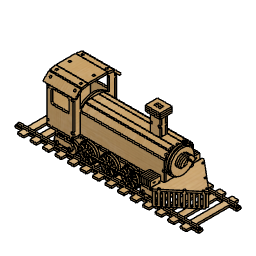
train-3D-model (Autodesk Fusion 360 design; units mm, degrees)
Autodesk Fusion 360 part; units mm, degrees
note: some values were not read from the file. Set by a fixed rule: which sketch regions a step uses.
(part 1 of 4)
sketch "Sketch1" plane through (0, 0, 0) normal (0, 1, 0) x (1, 0, 0)
  circle A0 centre (0, 0) radius 15
  line L0 (0, 0) -> (35, 0) construction
  circle A1 centre (35, 0) radius 15
  line L1 (0, 0) -> (-35, 0) construction
  circle A2 centre (-35, 0) radius 15
  line L2 (-33.5, -3) -> (-33.5, 3)
  line L3 (-33.5, 3) -> (-36.5, 3)
  line L4 (-36.5, 3) -> (-36.5, -3)
  line L5 (-36.5, -3) -> (-33.5, -3)
  line L6 (-1.5, -3) -> (-1.5, 3)
  line L7 (-1.5, 3) -> (1.5, 3)
  line L8 (1.5, 3) -> (1.5, -3)
  line L9 (1.5, -3) -> (-1.5, -3)
  line L10 (36.5, 3) -> (36.5, -3)
  line L11 (36.5, -3) -> (33.5, -3)
  line L12 (33.5, -3) -> (33.5, 3)
  line L13 (33.5, 3) -> (36.5, 3)
  circle A3 centre (81, 6) radius 9
  line L14 (35, 15) -> (81, 15) construction
  line L15 (35, 15) -> (61, 15) construction
  circle A4 centre (61, 6) radius 9
  line L16 (62.5, 3) -> (62.5, 9)
  line L17 (62.5, 9) -> (59.5, 9)
  line L18 (59.5, 9) -> (59.5, 3)
  line L19 (62.5, 3) -> (59.5, 3)
  line L20 (82.5, 3) -> (82.5, 9)
  line L21 (82.5, 9) -> (79.5, 9)
  line L22 (79.5, 9) -> (79.5, 3)
  line L23 (79.5, 3) -> (82.5, 3)
  circle A5 centre (-61, 6) radius 9
  circle A6 centre (-81, 6) radius 9
  line L24 (-62.5, 3) -> (-59.5, 3)
  line L25 (-59.5, 9) -> (-59.5, 3)
  line L26 (-62.5, 9) -> (-59.5, 9)
  line L27 (-62.5, 3) -> (-62.5, 9)
  line L28 (-79.5, 9) -> (-79.5, 3)
  line L29 (-79.5, 3) -> (-82.5, 3)
  line L30 (-82.5, 3) -> (-82.5, 9)
  line L31 (-82.5, 9) -> (-79.5, 9)
  dimension "d1" = 30
  dimension "d2" = 35
  dimension "d3" = 30
  dimension "d4" = 35
  dimension "d5" = 30
  dimension "d7" = 3
  dimension "d8" = 18
  dimension "d9" = 46
  dimension "d10" = 26
  dimension "d11" = 18
  dimension "d14" = 3
  dimension "d16" = 6
  dimension "d17" = 3
  constraint coincident A0.centre L0.start
  constraint horizontal L0
  constraint coincident L0.end A1.centre
  constraint parallel L0 L1
  constraint coincident L1.end A2.centre
  constraint perpendicular L1 L2
  constraint perpendicular L2 L3
  constraint perpendicular L3 L4
  constraint perpendicular L2 L5
  constraint coincident A1 L14.start
  constraint horizontal L14
  constraint tangent A1 L14
  constraint tangent A3 L14
  constraint coincident A3 L14.end
  constraint parallel L14 L15
  constraint tangent L15 A4
  constraint coincident L15.end A4
  constraint perpendicular L16 L17
  constraint perpendicular L17 L18
  constraint perpendicular L20 L21
  constraint perpendicular L21 L22
  constraint perpendicular L20 L23
  measures "d1" diameter of A0
  measures "d2" distance of A0.centre L0.end
  measures "d3" diameter of A1
  measures "d4" distance of A0.centre L1.end
  measures "d5" diameter of A2
  measures "d7" distance of L2.end L3.end
  measures "d8" diameter of A3
  measures "d9" distance of L14.start L14.end
  measures "d10" distance of L14.start L15.end
  measures "d11" diameter of A4
  measures "d14" distance of L16.end L17.end
  measures "d16" distance of L20.start L20.end
  measures "d17" distance of L20.end L21.end
extrude "Extrude1" add sketch "Sketch1" against normal blind 3 contours A6 makes body 1
extrude "Extrude2" add sketch "Sketch1" against normal blind 3 separate body contours A5 makes body 2
extrude "Extrude3" add sketch "Sketch1" against normal blind 3 separate body contours A2 makes body 3
extrude "Extrude4" add sketch "Sketch1" against normal blind 3 separate body contours A0 makes body 4
extrude "Extrude5" add sketch "Sketch1" against normal blind 3 separate body contours A1 makes body 5
extrude "Extrude6" add sketch "Sketch1" against normal blind 3 separate body contours A4 makes body 6
extrude "Extrude7" add sketch "Sketch1" against normal blind 3 separate body contours A3 makes body 7
ref_plane "WorkPlane1" through (-35, -3, 0) normal (0, -1, 0) x (-1, 0, 0)
sketch "Sketch2" plane through (0, -3, 0) normal (0, -1, 0) x (-1, 0, 0)
  line L0 (59.5, 9) -> (62.5, 9)
  line L1 (62.5, 9) -> (62.5, 3)
  line L2 (62.5, 3) -> (59.5, 3)
  line L3 (59.5, 3) -> (59.5, 9)
  line L4 (79.5, 9) -> (82.5, 9)
  line L5 (82.5, 9) -> (82.5, 3)
  line L6 (82.5, 3) -> (79.5, 3)
  line L7 (79.5, 3) -> (79.5, 9)
  line L8 (36.5, 3) -> (36.5, -3)
  line L9 (33.5, 3) -> (36.5, 3)
  line L10 (33.5, -3) -> (33.5, 3)
  line L11 (36.5, -3) -> (33.5, -3)
  line L12 (1.5, 3) -> (1.5, -3)
  line L13 (1.5, -3) -> (-1.5, -3)
  line L14 (-1.5, -3) -> (-1.5, 3)
  line L15 (-1.5, 3) -> (1.5, 3)
  line L16 (-33.5, 3) -> (-33.5, -3)
  line L17 (-33.5, -3) -> (-36.5, -3)
  line L18 (-36.5, -3) -> (-36.5, 3)
  line L19 (-36.5, 3) -> (-33.5, 3)
  line L20 (-62.5, 3) -> (-62.5, 9)
  line L21 (-62.5, 9) -> (-59.5, 9)
  line L22 (-59.5, 9) -> (-59.5, 3)
  line L23 (-59.5, 3) -> (-62.5, 3)
  line L24 (-79.5, 9) -> (-79.5, 3)
  line L25 (-79.5, 3) -> (-82.5, 3)
  line L26 (-82.5, 3) -> (-82.5, 9)
  line L27 (-82.5, 9) -> (-79.5, 9)
  circle A0 centre (81, 6) radius 8
  circle A1 centre (61, 6) radius 8
  circle A2 centre (35, 0) radius 14
  circle A3 centre (0, 0) radius 14
  circle A4 centre (-35, 0) radius 14
  circle A5 centre (-61, 6) radius 8
  circle A6 centre (-81, 6) radius 8
  line L28 (33.8353, -4.3467) -> (31.6354, -12.557)
  line L29 (36.1647, -4.3467) -> (38.3646, -12.557)
  line L30 (35, 0) -> (48, 0) construction
  arc A7 (31.6354, -12.557) -> (38.3646, -12.557) centre (35, 0) ccw
  arc A8 (33.8353, -4.3467) -> (36.1647, -4.3467) centre (35, 0) ccw
  line L31 (38.8971, -2.25) -> (46.2583, -6.5)
  arc A9 (41.5, -11.2583) -> (46.2583, -6.5) centre (35, 0) ccw
  line L32 (37.25, -3.8971) -> (41.5, -11.2583)
  arc A10 (37.25, -3.8971) -> (38.8971, -2.25) centre (35, 0) ccw
  line L33 (39.3467, 1.1647) -> (47.557, 3.3646)
  arc A11 (47.557, -3.3646) -> (47.557, 3.3646) centre (35, 0) ccw
  line L34 (39.3467, -1.1647) -> (47.557, -3.3646)
  arc A12 (39.3467, -1.1647) -> (39.3467, 1.1647) centre (35, 0) ccw
  line L35 (37.25, 3.8971) -> (41.5, 11.2583)
  arc A13 (46.2583, 6.5) -> (41.5, 11.2583) centre (35, 0) ccw
  line L36 (38.8971, 2.25) -> (46.2583, 6.5)
  arc A14 (38.8971, 2.25) -> (37.25, 3.8971) centre (35, 0) ccw
  line L37 (33.8353, 4.3467) -> (31.6354, 12.557)
  arc A15 (38.3646, 12.557) -> (31.6354, 12.557) centre (35, 0) ccw
  line L38 (36.1647, 4.3467) -> (38.3646, 12.557)
  arc A16 (36.1647, 4.3467) -> (33.8353, 4.3467) centre (35, 0) ccw
  line L39 (31.1029, 2.25) -> (23.7417, 6.5)
  arc A17 (28.5, 11.2583) -> (23.7417, 6.5) centre (35, 0) ccw
  line L40 (32.75, 3.8971) -> (28.5, 11.2583)
  arc A18 (32.75, 3.8971) -> (31.1029, 2.25) centre (35, 0) ccw
  line L41 (30.6533, -1.1647) -> (22.443, -3.3646)
  arc A19 (22.443, 3.3646) -> (22.443, -3.3646) centre (35, 0) ccw
  line L42 (30.6533, 1.1647) -> (22.443, 3.3646)
  arc A20 (30.6533, 1.1647) -> (30.6533, -1.1647) centre (35, 0) ccw
  line L43 (32.75, -3.8971) -> (28.5, -11.2583)
  arc A21 (23.7417, -6.5) -> (28.5, -11.2583) centre (35, 0) ccw
  line L44 (31.1029, -2.25) -> (23.7417, -6.5)
  arc A22 (31.1029, -2.25) -> (32.75, -3.8971) centre (35, 0) ccw
  arc A23 (-2.25, 3.8971) -> (-3.8971, 2.25) centre (0, 0) ccw
  arc A24 (4.3467, -1.1647) -> (4.3467, 1.1647) centre (0, 0) ccw
  arc A25 (-3.8971, -2.25) -> (-2.25, -3.8971) centre (0, 0) ccw
  line L45 (-3.8971, -2.25) -> (-11.2583, -6.5)
  line L46 (2.25, 3.8971) -> (6.5, 11.2583)
  line L47 (-2.25, -3.8971) -> (-6.5, -11.2583)
  arc A26 (-6.5, 11.2583) -> (-11.2583, 6.5) centre (0, 0) ccw
  arc A27 (-12.557, 3.3646) -> (-12.557, -3.3646) centre (0, 0) ccw
  arc A28 (12.557, -3.3646) -> (12.557, 3.3646) centre (0, 0) ccw
  arc A29 (1.1647, 4.3467) -> (-1.1647, 4.3467) centre (0, 0) ccw
  line L48 (-3.8971, 2.25) -> (-11.2583, 6.5)
  arc A30 (-1.1647, -4.3467) -> (1.1647, -4.3467) centre (0, 0) ccw
  arc A31 (2.25, -3.8971) -> (3.8971, -2.25) centre (0, 0) ccw
  line L49 (1.1647, -4.3467) -> (3.3646, -12.557)
  arc A32 (11.2583, 6.5) -> (6.5, 11.2583) centre (0, 0) ccw
  arc A33 (-4.3467, 1.1647) -> (-4.3467, -1.1647) centre (0, 0) ccw
  line L50 (-1.1647, -4.3467) -> (-3.3646, -12.557)
  arc A34 (3.3646, 12.557) -> (-3.3646, 12.557) centre (0, 0) ccw
  line L51 (3.8971, 2.25) -> (11.2583, 6.5)
  line L52 (1.1647, 4.3467) -> (3.3646, 12.557)
  line L53 (4.3467, 1.1647) -> (12.557, 3.3646)
  arc A35 (3.8971, 2.25) -> (2.25, 3.8971) centre (0, 0) ccw
  line L54 (2.25, -3.8971) -> (6.5, -11.2583)
  line L55 (-2.25, 3.8971) -> (-6.5, 11.2583)
  circle A36 centre (0, 0) radius 14
  line L56 (0, 0) -> (-13, 0) construction
  line L57 (-4.3467, 1.1647) -> (-12.557, 3.3646)
  arc A37 (-3.3646, -12.557) -> (3.3646, -12.557) centre (0, 0) ccw
  line L58 (3.8971, -2.25) -> (11.2583, -6.5)
  line L59 (4.3467, -1.1647) -> (12.557, -3.3646)
  arc A38 (6.5, -11.2583) -> (11.2583, -6.5) centre (0, 0) ccw
  line L60 (-1.1647, 4.3467) -> (-3.3646, 12.557)
  arc A39 (-11.2583, -6.5) -> (-6.5, -11.2583) centre (0, 0) ccw
  line L61 (-4.3467, -1.1647) -> (-12.557, -3.3646)
  arc A40 (-23.7417, 6.5) -> (-28.5, 11.2583) centre (-35, 0) ccw
  line L62 (-38.8971, 2.25) -> (-46.2583, 6.5)
  circle A41 centre (-35, 0) radius 14
  line L63 (-39.3467, 1.1647) -> (-47.557, 3.3646)
  line L64 (-30.6533, -1.1647) -> (-22.443, -3.3646)
  line L65 (-35, 0) -> (-48, 0) construction
  line L66 (-39.3467, -1.1647) -> (-47.557, -3.3646)
  line L67 (-33.8353, 4.3467) -> (-31.6354, 12.557)
  arc A42 (-32.75, -3.8971) -> (-31.1029, -2.25) centre (-35, 0) ccw
  arc A43 (-41.5, 11.2583) -> (-46.2583, 6.5) centre (-35, 0) ccw
  arc A44 (-31.6354, 12.557) -> (-38.3646, 12.557) centre (-35, 0) ccw
  arc A45 (-39.3467, 1.1647) -> (-39.3467, -1.1647) centre (-35, 0) ccw
  line L68 (-37.25, 3.8971) -> (-41.5, 11.2583)
  arc A46 (-36.1647, -4.3467) -> (-33.8353, -4.3467) centre (-35, 0) ccw
  arc A47 (-46.2583, -6.5) -> (-41.5, -11.2583) centre (-35, 0) ccw
  arc A48 (-31.1029, 2.25) -> (-32.75, 3.8971) centre (-35, 0) ccw
  arc A49 (-22.443, -3.3646) -> (-22.443, 3.3646) centre (-35, 0) ccw
  line L69 (-32.75, 3.8971) -> (-28.5, 11.2583)
  arc A50 (-38.3646, -12.557) -> (-31.6354, -12.557) centre (-35, 0) ccw
  line L70 (-37.25, -3.8971) -> (-41.5, -11.2583)
  line L71 (-36.1647, 4.3467) -> (-38.3646, 12.557)
  arc A51 (-38.8971, -2.25) -> (-37.25, -3.8971) centre (-35, 0) ccw
  line L72 (-32.75, -3.8971) -> (-28.5, -11.2583)
  arc A52 (-30.6533, -1.1647) -> (-30.6533, 1.1647) centre (-35, 0) ccw
  arc A53 (-28.5, -11.2583) -> (-23.7417, -6.5) centre (-35, 0) ccw
  line L73 (-36.1647, -4.3467) -> (-38.3646, -12.557)
  line L74 (-31.1029, 2.25) -> (-23.7417, 6.5)
  line L75 (-38.8971, -2.25) -> (-46.2583, -6.5)
  line L76 (-33.8353, -4.3467) -> (-31.6354, -12.557)
  arc A54 (-37.25, 3.8971) -> (-38.8971, 2.25) centre (-35, 0) ccw
  arc A55 (-47.557, 3.3646) -> (-47.557, -3.3646) centre (-35, 0) ccw
  arc A56 (-33.8353, 4.3467) -> (-36.1647, 4.3467) centre (-35, 0) ccw
  line L77 (-31.1029, -2.25) -> (-23.7417, -6.5)
  line L78 (-30.6533, 1.1647) -> (-22.443, 3.3646)
  point P0 (-1.5, -3)
  point P1 (-1.5, 3)
  point P2 (1.5, -3)
  point P3 (1.5, 3)
  dimension "d33" = 16
  dimension "d34" = 16
  dimension "d35" = 28
  dimension "d36" = 28
  dimension "d37" = 28
  dimension "d38" = 16
  dimension "d39" = 16
  dimension "d40" = 9
  dimension "d41" = 26
  dimension "d43" = 75
  dimension "d45" = 360
  constraint coincident A3.centre A23.centre
  constraint concentric A2 A8
  constraint concentric A7 A8
  constraint horizontal L30
  constraint coincident A2.centre L30.start
  measures "d33" diameter of A0
  measures "d34" diameter of A1
  measures "d35" diameter of A2
  measures "d36" diameter of A3
  measures "d37" diameter of A4
  measures "d38" diameter of A5
  measures "d39" diameter of A6
  measures "d40" diameter of A8
  measures "d41" diameter of A7
  measures "d43" angle of L29 L30
extrude "Extrude8" add sketch "Sketch2" along normal blind 3 separate body contours A0 makes body 8
extrude "Extrude9" add sketch "Sketch2" along normal blind 3 separate body contours A1 makes body 9
extrude "Extrude10" add sketch "Sketch2" along normal blind 3 separate body contours A2 makes body 10
extrude "Extrude11" add sketch "Sketch2" along normal blind 3 separate body contours A3 A36 makes body 11
extrude "Extrude12" add sketch "Sketch2" along normal blind 3 separate body contours A4 A41 makes body 12
extrude "Extrude13" add sketch "Sketch2" along normal blind 3 separate body contours A5 makes body 13
extrude "Extrude14" add sketch "Sketch2" along normal blind 3 separate body contours A6 makes body 14
ref_plane "WorkPlane2" through (-35, -6, 0) normal (0, -1, 0) x (-1, 0, 0)
sketch "Sketch3" plane through (0, -6, 0) normal (0, -1, 0) x (-1, 0, 0)
  line L0 (82.5, 3) -> (79.5, 3)
  line L1 (62.5, 3) -> (59.5, 3)
  line L2 (-59.5, 3) -> (-62.5, 3)
  line L3 (-79.5, 3) -> (-82.5, 3)
  line L4 (33.9625, -5.5834) -> (30.7825, -2.3055)
  arc A0 (33.9625, -5.5834) -> (36.611, -0.5356) centre (36.1157, -3.4944) ccw
  arc A1 (32.1068, 0.2184) -> (30.38, -1.0114) centre (31.8591, -1.261) ccw
  line L5 (33.5, -3) -> (33.5, -0.0149)
  line L6 (36.5, -3) -> (36.5, -0.517)
  line L7 (33.5, -3) -> (36.5, -3)
  line L8 (36.611, -0.5356) -> (36.5, -0.517)
  line L9 (33.5, -0.0149) -> (32.1068, 0.2184)
  line L10 (1.5, -2.9851) -> (1.5, -0.5022)
  line L11 (-1.5, -2.9851) -> (1.5, -2.9851)
  line L12 (-1.5, 0) -> (-2.8932, 0.2332)
  arc A2 (-2.8932, 0.2332) -> (-4.6224, -1.0114) centre (-3.1409, -1.2462) ccw
  line L13 (-1.5, -2.9851) -> (-1.5, 0)
  line L14 (-1.0375, -5.5685) -> (-4.2175, -2.2907)
  line L15 (1.611, -0.5208) -> (1.5, -0.5022)
  line L16 (-36.5, -2.9851) -> (-33.5, -2.9851)
  line L17 (-33.389, -0.5208) -> (-33.5, -0.5022)
  line L18 (-33.5, -2.9851) -> (-33.5, -0.5022)
  line L19 (-36.5, -2.9851) -> (-36.5, 0)
  arc A3 (-37.8932, 0.2332) -> (-39.2175, -2.2907) centre (-38.1409, -1.2462) ccw
  line L20 (-36.0375, -5.5685) -> (-38.2212, -3.3176)
  line L21 (-36.5, 0) -> (-37.8932, 0.2332)
  line L22 (30.7825, -2.3055) -> (3.8764, -2.3055)
  line L23 (30.38, -1.0114) -> (2.821, -1.0114)
  arc A4 (-1.0375, -5.5685) -> (3.8764, -2.3055) centre (1.1157, -3.4796) ccw
  arc A5 (2.821, -1.0114) -> (1.611, -0.5208) centre (1.1157, -3.4796) ccw
  line L24 (-4.2031, -2.3055) -> (-31.1236, -2.3055)
  line L25 (-4.6224, -1.0114) -> (-32.179, -1.0114)
  arc A6 (-36.0375, -5.5685) -> (-31.1236, -2.3055) centre (-33.8843, -3.4796) ccw
  arc A7 (-32.179, -1.0114) -> (-33.389, -0.5208) centre (-33.8843, -3.4796) ccw
  line L26 (-59.5, 6) -> (-57.5, 6)
  line L27 (-82.5, 6) -> (-84.5, 6)
  line L28 (-56.5, 5) -> (-56.5, 0)
  line L29 (-59.5, -3) -> (-82.5, -3)
  line L30 (-85.5, 0) -> (-85.5, 5)
  line L31 (-62.5, 6) -> (-79.5, 6)
  arc A8 (-59.5, -3) -> (-56.5, 0) centre (-59.5, 0) ccw
  arc A9 (-85.5, 0) -> (-82.5, -3) centre (-82.5, 0) ccw
  arc A10 (-56.5, 5) -> (-57.5, 6) centre (-57.5, 5) ccw
  arc A11 (-84.5, 6) -> (-85.5, 5) centre (-84.5, 5) ccw
  line L32 (79.5, 6) -> (62.5, 6)
  line L33 (82.5, 6) -> (84.5, 6)
  line L34 (59.5, 6) -> (57.5, 6)
  line L35 (85.5, 5) -> (85.5, 0)
  line L36 (82.5, -3) -> (59.5, -3)
  line L37 (56.5, 0) -> (56.5, 5)
  arc A12 (82.5, -3) -> (85.5, 0) centre (82.5, 0) ccw
  arc A13 (56.5, 0) -> (59.5, -3) centre (59.5, 0) ccw
  arc A14 (85.5, 5) -> (84.5, 6) centre (84.5, 5) ccw
  arc A15 (57.5, 6) -> (56.5, 5) centre (57.5, 5) ccw
  line L38 (-39.2175, -2.2907) -> (-44, -15)
  line L39 (-38.2212, -3.3176) -> (-42.5217, -14.7459)
  arc A16 (-44.7585, -16.2941) -> (-42.5217, -14.7459) centre (-44, -15) ccw
  line L40 (-79.5, 3) -> (-79.5, 6)
  line L41 (-82.5, 3) -> (-82.5, 6)
  line L42 (-62.5, 3) -> (-62.5, 6)
  line L43 (-59.5, 3) -> (-59.5, 6)
  line L44 (59.5, 3) -> (59.5, 6)
  line L45 (62.5, 3) -> (62.5, 6)
  line L46 (79.5, 3) -> (79.5, 6)
  line L47 (82.5, 3) -> (82.5, 6)
  line L48 (-78, -15) -> (-78, -16.2941)
  line L49 (-44.7585, -16.2941) -> (-78, -16.2941)
  line L50 (-44, -15) -> (-78, -15)
  point P0 (-1.5, 0)
  point P1 (-36.5, 0)
  point P2 (-56.5, 6)
  point P3 (-85.5, 6)
  point P4 (85.5, 6)
  point P5 (56.5, 6)
  dimension "d76" = 6
  dimension "d77" = 3
  dimension "d78" = 6
  dimension "d79" = 3
  dimension "d80" = 6
  dimension "d83" = 3
  dimension "d84" = 3
  dimension "d85" = 3
  dimension "d86" = 1
  dimension "d87" = 1
  dimension "d88" = 3
  dimension "d89" = 3
  dimension "d90" = 3
  dimension "d91" = 3
  dimension "d92" = 1
  dimension "d93" = 1
  dimension "d94" = 1.2941
  dimension "d97" = 1.2941
  dimension "d99" = 3
  constraint tangent L4 A1
  constraint tangent A1 L8
  constraint tangent L4 A0
  constraint tangent A0 L8
  constraint perpendicular L6 L7
  constraint coincident L5.end L8
  constraint collinear L8 L9
  constraint tangent A2 L14
  constraint tangent A2 L15
  constraint tangent L14 A4
  constraint tangent L15 A4
  constraint perpendicular L10 L11
  constraint coincident P0 L15
  constraint collinear L12 L15
  constraint tangent A3 L20
  constraint tangent L17 A3
  constraint tangent L20 A6
  constraint tangent L17 A6
  constraint perpendicular L16 L18
  constraint coincident P1 L17
  constraint collinear L17 L21
  constraint horizontal L22
  constraint horizontal L23
  constraint coincident L23.end A4
  constraint concentric A4 A5
  constraint coincident L14 L24.start
  constraint coincident L25.end A6
  constraint parallel L23 L25
  constraint concentric A6 A7
  constraint perpendicular L26 L28
  constraint perpendicular L28 L29
  constraint perpendicular L29 L30
  constraint tangent L28 A8
  constraint tangent L29 A8
  constraint tangent L29 A9
  constraint tangent L30 A9
  constraint coincident P2 L28
  constraint coincident P2 L26
  constraint tangent L28 A10
  constraint tangent L26 A10
  constraint coincident P3 L27
  constraint coincident P3 L30
  constraint tangent L27 A11
  constraint tangent L30 A11
  constraint perpendicular L33 L35
  constraint perpendicular L35 L36
  constraint perpendicular L34 L37
  constraint tangent L35 A12
  constraint tangent L36 A12
  constraint tangent L36 A13
  constraint tangent L37 A13
  constraint coincident P4 L35
  constraint coincident P4 L33
  constraint tangent L35 A14
  constraint tangent L33 A14
  constraint coincident P5 L34
  constraint coincident P5 L37
  constraint tangent L34 A15
  constraint tangent L37 A15
  constraint coincident L38.end A16.centre
  constraint coincident L3.start L40.start
  constraint vertical L40
  constraint coincident L3.end L41.start
  constraint perpendicular L27 L41
  constraint coincident L2.end L42.start
  constraint vertical L42
  constraint coincident L2.start L43.start
  constraint perpendicular L26 L43
  constraint coincident L1.end L44.start
  constraint perpendicular L34 L44
  constraint coincident L1.start L45.start
  constraint parallel L44 L45
  constraint coincident L0.end L46.start
  constraint vertical L46
  constraint coincident L0.start L47.start
  constraint perpendicular L33 L47
  measures "d76" diameter of A0
  measures "d77" diameter of A1
  measures "d78" diameter of A4
  measures "d79" diameter of A2
  measures "d80" diameter of A6
  measures "d83" distance of L27.start P3
  measures "d84" radius of A8
  measures "d85" radius of A9
  measures "d86" radius of A10
  measures "d87" radius of A11
  measures "d88" distance of L33.start P4
  measures "d89" distance of L34.start P5
  measures "d90" radius of A12
  measures "d91" radius of A13
  measures "d92" radius of A14
  measures "d93" radius of A15
  measures "d94" distance of L22 L23
  measures "d97" distance of L24 L25
  measures "d99" diameter of A16
extrude "Extrude15" add sketch "Sketch3" along normal blind 3 separate body contours L0 L1 L32 L33 L34 L35 L36 L37 A12 A13 A14 A15 L44 L45 L46 L47 makes body 15
extrude "Extrude16" add sketch "Sketch3" along normal blind 3 separate body contours L4 A0 A1 L5 L6 L7 L8 L9 L10 L11 L12 A2 L13 L14 L15 L16 L17 L18 L19 A3 L20 L21 L22 L23 A4 A5 L24 L25 A6 A7 L38 L39 A16 L48 L49 L50 makes body 16
extrude "Extrude17" add sketch "Sketch3" along normal blind 3 separate body contours L2 L3 L26 L27 L28 L29 L30 L31 A8 A9 A10 A11 L40 L41 L42 L43 makes body 17
ref_plane "WorkPlane3" through (35, 3, 0) normal (0, -1, 0) x (-1, 0, 0)
sketch "Sketch4" plane through (0, 3, 0) normal (0, -1, 0) x (-1, 0, 0)
  line L0 (93, -10) -> (93, 5)
  line L1 (82.5, 9) -> (82.5, 3)
  line L2 (82.5, 3) -> (79.5, 3)
  line L3 (79.5, 3) -> (79.5, 9)
  line L4 (79.5, 9) -> (82.5, 9)
  line L5 (62.5, 9) -> (62.5, 3)
  line L6 (59.5, 9) -> (62.5, 9)
  line L7 (59.5, 3) -> (59.5, 9)
  line L8 (62.5, 3) -> (59.5, 3)
  line L9 (36.5, 3) -> (36.5, -3)
  line L10 (36.5, -3) -> (33.5, -3)
  line L11 (33.5, -3) -> (33.5, 3)
  line L12 (33.5, 3) -> (36.5, 3)
  line L13 (1.5, 3) -> (1.5, -3)
  line L14 (-1.5, 3) -> (1.5, 3)
  line L15 (-1.5, -3) -> (-1.5, 3)
  line L16 (1.5, -2.9851) -> (-1.5, -2.9851)
  line L17 (-33.5, 3) -> (-33.5, -3)
  line L18 (-36.5, 3) -> (-33.5, 3)
  line L19 (-36.5, -3) -> (-36.5, 3)
  line L20 (-33.5, -2.9851) -> (-36.5, -2.9851)
  line L21 (-59.5, 9) -> (-59.5, 3)
  line L22 (-62.5, 3) -> (-62.5, 9)
  line L23 (-59.5, 3) -> (-62.5, 3)
  line L24 (-79.5, 9) -> (-79.5, 3)
  line L25 (-82.5, 9) -> (-79.5, 9)
  line L26 (-82.5, 3) -> (-82.5, 9)
  line L27 (-79.5, 3) -> (-82.5, 3)
  line L28 (80, -10) -> (80, -13)
  line L29 (80, -13) -> (77.75, -13)
  line L30 (77, -12.25) -> (77, -10)
  line L31 (77, -10) -> (51, -10)
  line L32 (51, -10) -> (51, -13)
  line L33 (51, -13) -> (48, -13)
  line L34 (48, -13) -> (48, -10)
  line L35 (48, -10) -> (22, -10)
  line L36 (22, -10) -> (22, -13)
  line L37 (22, -13) -> (19, -13)
  line L38 (19, -13) -> (19, -10)
  line L39 (19, -10) -> (-7, -10)
  line L40 (-7, -10) -> (-7, -13)
  line L41 (-7, -13) -> (-10, -13)
  line L42 (-10, -13) -> (-10, -10)
  line L43 (-10, -10) -> (-36, -10)
  line L44 (-36, -10) -> (-36, -13)
  line L45 (-36, -13) -> (-39, -13)
  line L46 (-39, -13) -> (-39, -10)
  line L47 (-39, -10) -> (-65, -10)
  line L48 (-65, -10) -> (-65, -13)
  line L49 (-65, -13) -> (-68, -13)
  line L50 (-68, -13) -> (-68, -10)
  line L51 (-68, -10) -> (-84, -10)
  line L52 (93, -10) -> (80, -10)
  line L53 (-82.5, 9) -> (-82.5, 3)
  line L54 (-82.5, 3) -> (-79.5, 3)
  line L55 (-79.5, 3) -> (-79.5, 9)
  line L56 (-79.5, 9) -> (-82.5, 9)
  arc A0 (77, -12.25) -> (77.75, -13) centre (77.75, -12.25) ccw
  arc A1 (93, 5) -> (88, 10) centre (88, 5) ccw
  line L57 (88, 4.5) -> (85, 4.5)
  line L58 (88, 1.5) -> (85, 1.5)
  line L59 (85, 1.5) -> (85, 4.5)
  line L60 (88, 4.5) -> (88, 1.5)
  line L61 (-84, 1.5) -> (-87, 1.5)
  line L62 (-84, -1.5) -> (-87, -1.5)
  line L63 (-87, 1.5) -> (-87, -1.5)
  line L64 (-84, -10) -> (-84, -1.5)
  line L65 (-84, 1.5) -> (-84, 10)
  line L66 (88, 10) -> (-84, 10)
  line L67 (-59.5, 9) -> (-62.5, 9)
  point P0 (93, 10)
  point P1 (77, -13)
  dimension "d108" = 177
  dimension "d111" = 3
  dimension "d112" = 26
  dimension "d158" = 0.75
  dimension "d159" = 5
  constraint perpendicular L28 L29
  constraint perpendicular L29 L30
  constraint perpendicular L30 L31
  constraint perpendicular L31 L32
  constraint perpendicular L32 L33
  constraint perpendicular L33 L34
  constraint perpendicular L34 L35
  constraint perpendicular L35 L36
  constraint perpendicular L36 L37
  constraint perpendicular L37 L38
  constraint perpendicular L38 L39
  constraint perpendicular L39 L40
  constraint perpendicular L40 L41
  constraint perpendicular L41 L42
  constraint perpendicular L42 L43
  constraint perpendicular L43 L44
  constraint perpendicular L44 L45
  constraint perpendicular L45 L46
  constraint perpendicular L44 L47
  constraint perpendicular L47 L48
  constraint perpendicular L48 L49
  constraint perpendicular L49 L50
  constraint perpendicular L51 L64
  constraint perpendicular L28 L52
  constraint coincident P1 L29
  constraint coincident P1 L30
  constraint tangent L29 A0
  constraint tangent L30 A0
  constraint coincident P0 L0
  constraint tangent L0 A1
  constraint perpendicular L57 L59
  constraint perpendicular L58 L60
  constraint perpendicular L62 L63
  constraint collinear L64 L65
  constraint tangent A1 L66
  constraint coincident L21.start L67.start
  constraint coincident L22.end L67.end
  measures "d108" distance of P0 L65.end
  measures "d111" distance of L28.end P1
  measures "d112" distance of L30.end L31.end
  measures "d158" radius of A0
  measures "d159" radius of A1
extrude "Extrude18" add sketch "Sketch4" along normal blind 3 separate body makes body 18
ref_plane "WorkPlane4" through (-64, 1.5, 10) normal (0, 0, 1) x (-1, 0, 0)
sketch "Sketch5" plane through (0, 0, 10) normal (0, 0, 1) x (1, 0, 0)
  line L0 (-80, 3) -> (-80, 0)
  line L1 (-80, 51) -> (-80, 54)
  line L2 (-80, 51) -> (-77, 51)
  line L3 (-77, 51) -> (-77, 54)
  line L4 (-77, 54) -> (-80, 54)
  line L5 (-51, 3) -> (-51, 0)
  line L6 (-51, 3) -> (-48, 3)
  line L7 (-48, 3) -> (-48, 0)
  line L8 (-22, 3) -> (-22, 0)
  line L9 (-22, 3) -> (-19, 3)
  line L10 (-19, 3) -> (-19, 0)
  line L11 (7, 3) -> (7, 0)
  line L12 (7, 3) -> (10, 3)
  line L13 (10, 3) -> (10, 0)
  line L14 (36, 3) -> (36, 0)
  line L15 (36, 3) -> (39, 3)
  line L16 (39, 3) -> (39, 0)
  line L17 (65, 3) -> (65, 0)
  line L18 (65, 3) -> (68, 3)
  line L19 (68, 3) -> (68, 0)
  line L20 (-51, 0) -> (-55, 0)
  line L21 (-22, 0) -> (-48, 0)
  line L22 (7, 0) -> (-19, 0)
  line L23 (36, 0) -> (10, 0)
  line L24 (65, 0) -> (39, 0)
  line L25 (68, 0) -> (80.2343, 0)
  line L26 (7, 54) -> (-19, 54)
  line L27 (10, 51) -> (10, 54)
  line L28 (7, 51) -> (7, 54)
  line L29 (36, 54) -> (10, 54)
  line L30 (36, 51) -> (39, 51)
  line L31 (68, 51) -> (68, 54)
  line L32 (65, 51) -> (68, 51)
  line L33 (-22, 51) -> (-22, 54)
  line L34 (65, 54) -> (39, 54)
  line L35 (36, 51) -> (36, 54)
  line L36 (68, 54) -> (80.2343, 54)
  line L37 (39, 51) -> (39, 54)
  line L38 (-22, 51) -> (-19, 51)
  line L39 (7, 51) -> (10, 51)
  line L40 (65, 51) -> (65, 54)
  line L41 (-19, 51) -> (-19, 54)
  line L42 (-22, 54) -> (-48, 54)
  line L43 (-48, 51) -> (-48, 54)
  line L44 (-51, 51) -> (-48, 51)
  line L45 (-51, 51) -> (-51, 54)
  line L46 (-51, 54) -> (-55, 54)
  line L47 (-55, 63) -> (-55, 54)
  line L48 (-55, 0) -> (-55, -9)
  line L49 (-98, -9) -> (-93, -9)
  line L50 (-93, -9) -> (-93, -6)
  line L51 (-93, -6) -> (-90, -6)
  line L52 (-90, -6) -> (-90, -9)
  line L53 (-55, -9) -> (-58, -9)
  line L54 (-58, -9) -> (-58, -6)
  line L55 (-58, -6) -> (-61, -6)
  line L56 (-61, -6) -> (-61, -9)
  line L57 (-90, -9) -> (-61, -9)
  line L58 (-98, 63) -> (-93, 63)
  line L59 (-93, 63) -> (-93, 60)
  line L60 (-93, 60) -> (-90, 60)
  line L61 (-90, 60) -> (-90, 63)
  line L62 (-98, 63) -> (-98, 58)
  line L63 (-98, 58) -> (-95, 58)
  line L64 (-95, 58) -> (-95, 55)
  line L65 (-95, 55) -> (-98, 55)
  line L66 (-98, -9) -> (-98, -4)
  line L67 (-98, -4) -> (-95, -4)
  line L68 (-95, -4) -> (-95, -1)
  line L69 (-95, -1) -> (-98, -1)
  line L70 (-98, -1) -> (-98, 25.5)
  line L71 (-98, 55) -> (-98, 28.5)
  line L72 (-98, 28.5) -> (-95, 28.5)
  line L73 (-98, 25.5) -> (-95, 25.5)
  line L74 (-95, 25.5) -> (-95, 28.5)
  line L75 (-55, 46) -> (-58, 46)
  line L76 (-55, 46) -> (-55, 43)
  line L77 (-55, 43) -> (-58, 43)
  line L78 (-58, 46) -> (-58, 43)
  line L79 (-55, 8) -> (-58, 8)
  line L80 (-58, 8) -> (-58, 11)
  line L81 (-58, 11) -> (-55, 11)
  line L82 (-55, 11) -> (-55, 8)
  line L83 (-36.5, 3) -> (-33.5, 3)
  line L84 (-33.5, 3) -> (-33.5, 6)
  line L85 (-33.5, 6) -> (-36.5, 6)
  line L86 (-36.5, 6) -> (-36.5, 3)
  line L87 (-7.5, 3) -> (-4.5, 3)
  line L88 (21.5, 3) -> (24.5, 3)
  line L89 (50.5, 3) -> (53.5, 3)
  line L90 (-7.5, 3) -> (-7.5, 6)
  line L91 (-7.5, 6) -> (-4.5, 6)
  line L92 (-4.5, 6) -> (-4.5, 3)
  line L93 (24.5, 3) -> (24.5, 6)
  line L94 (24.5, 6) -> (21.5, 6)
  line L95 (21.5, 6) -> (21.5, 3)
  line L96 (50.5, 3) -> (50.5, 6)
  line L97 (50.5, 6) -> (53.5, 6)
  line L98 (53.5, 6) -> (53.5, 3)
  line L99 (-7.5, 51) -> (-7.5, 48)
  line L100 (-7.5, 51) -> (-4.5, 51)
  line L101 (-4.5, 48) -> (-4.5, 51)
  line L102 (-7.5, 48) -> (-4.5, 48)
  line L103 (-33.5, 51) -> (-33.5, 48)
  line L104 (-36.5, 51) -> (-33.5, 51)
  line L105 (-36.5, 48) -> (-36.5, 51)
  line L106 (-33.5, 48) -> (-36.5, 48)
  line L107 (21.5, 48) -> (21.5, 51)
  line L108 (24.5, 48) -> (21.5, 48)
  line L109 (24.5, 51) -> (24.5, 48)
  line L110 (21.5, 51) -> (24.5, 51)
  line L111 (50.5, 51) -> (50.5, 48)
  line L112 (50.5, 48) -> (53.5, 48)
  line L113 (53.5, 48) -> (53.5, 51)
  line L114 (50.5, 51) -> (53.5, 51)
  line L115 (-80, 0) -> (-77, 0)
  line L116 (-77, 0) -> (-77, 3)
  line L117 (-77, 3) -> (-80, 3)
  line L118 (81, 28.5) -> (81, 25.5)
  line L119 (81, 28.5) -> (84, 28.5)
  line L120 (81, 25.5) -> (84, 25.5)
  line L121 (84, 28.5) -> (84, 25.5)
  line L122 (87.8285, -11.784) -> (85.8989, -9.4869)
  line L123 (85.8989, -9.4869) -> (88.1961, -7.5573)
  line L124 (88.1961, -7.5573) -> (90.1256, -9.8545)
  line L125 (87.8285, 65.784) -> (85.8989, 63.4869)
  line L126 (85.8989, 63.4869) -> (88.1961, 61.5573)
  line L127 (88.1961, 61.5573) -> (90.1256, 63.8545)
  line L128 (130.1715, 30.216) -> (128.2419, 27.9188)
  line L129 (128.2419, 27.9188) -> (125.9448, 29.8484)
  line L130 (125.9448, 29.8484) -> (127.8744, 32.1455)
  line L131 (130.1715, 30.216) -> (134, 27)
  line L132 (130.1715, 23.784) -> (128.2419, 26.0812)
  line L133 (128.2419, 26.0812) -> (125.9448, 24.1516)
  line L134 (125.9448, 24.1516) -> (127.8744, 21.8545)
  line L135 (130.1715, 23.784) -> (134, 27)
  line L136 (108.9847, 9.9051) -> (111.2818, 11.8347)
  line L137 (111.2818, 11.8347) -> (113.2114, 9.5376)
  line L138 (108.9847, 9.9051) -> (110.9143, 7.608)
  line L139 (90.1256, -9.8545) -> (110.9143, 7.608)
  line L140 (113.2114, 9.5376) -> (127.8744, 21.8545)
  line L141 (111.2818, 42.1653) -> (113.2114, 44.4624)
  line L142 (108.9847, 44.0949) -> (110.9143, 46.392)
  line L143 (111.2818, 42.1653) -> (108.9847, 44.0949)
  line L144 (90.1256, 63.8545) -> (110.9143, 46.392)
  line L145 (113.2114, 44.4624) -> (127.8744, 32.1455)
  line L146 (87.8285, -11.784) -> (83.2343, -15.6432)
  line L147 (83.2343, -15.6432) -> (80.2343, -15.6432)
  line L148 (80.2343, -15.6432) -> (80.2343, 0)
  line L149 (87.8285, 65.784) -> (83.2343, 69.6432)
  line L150 (83.2343, 69.6432) -> (80.2343, 69.6432)
  line L151 (80.2343, 69.6432) -> (80.2343, 54)
  line L152 (-88, 45) -> (-85, 45)
  line L153 (-85, 45) -> (-85, 42)
  line L154 (-85, 42) -> (-88, 42)
  line L155 (-88, 42) -> (-88, 45)
  line L156 (-88, 9) -> (-85, 9)
  line L157 (-85, 9) -> (-85, 12)
  line L158 (-85, 12) -> (-88, 12)
  line L159 (-88, 12) -> (-88, 9)
  line L160 (-55, 63) -> (-58, 63)
  line L161 (-58, 63) -> (-58, 60)
  line L162 (-58, 60) -> (-61, 60)
  line L163 (-61, 60) -> (-61, 63)
  line L164 (-61, 63) -> (-90, 63)
  point P0 (0, 54)
  dimension "d170" = 3
  dimension "d171" = 3
  dimension "d172" = 3
  dimension "d173" = 3
  dimension "d174" = 3
  dimension "d176" = 5
  dimension "d177" = 3
  dimension "d215" = 5
  dimension "d216" = 5
  dimension "d217" = 3
  dimension "d218" = 3
  dimension "d219" = 26.5
  dimension "d220" = 26.5
  dimension "d256" = 3
  dimension "d257" = 90
  dimension "d258" = 3
  dimension "d259" = 3
  dimension "d260" = 3
  dimension "d261" = 3
  dimension "d313" = 3
  dimension "d314" = 3
  dimension "d315" = 3
  dimension "d316" = 3
  dimension "d317" = 3
  dimension "d402" = 3
  dimension "d522" = 3
  dimension "d523" = 3
  dimension "d525" = 3
  dimension "d526" = 3
  dimension "d529" = 5
  dimension "d530" = 5
  dimension "d531" = 3
  dimension "d532" = 3
  dimension "d533" = 3
  dimension "d534" = 3
  dimension "d535" = 3
  dimension "d536" = 3
  dimension "d539" = -3
  dimension "d579" = 6
  dimension "d580" = 3
  dimension "d581" = 6
  dimension "d582" = 3
  dimension "d764" = 3
  dimension "d765" = 3
  dimension "d766" = 3
  dimension "d767" = 3
  constraint coincident L5.end L20.start
  constraint coincident L8.end L21.start
  constraint coincident L7.end L21.end
  constraint coincident L11.end L22.start
  constraint coincident L10.end L22.end
  constraint coincident L14.end L23.start
  constraint coincident L13.end L23.end
  constraint coincident L17.end L24.start
  constraint coincident L16.end L24.end
  constraint coincident L19.end L25.start
  constraint perpendicular L49 L50
  constraint perpendicular L50 L51
  constraint perpendicular L51 L52
  constraint perpendicular L48 L53
  constraint perpendicular L53 L54
  constraint perpendicular L54 L55
  constraint perpendicular L55 L56
  constraint perpendicular L58 L59
  constraint perpendicular L59 L60
  constraint perpendicular L60 L61
  constraint perpendicular L58 L62
  constraint perpendicular L62 L63
  constraint perpendicular L63 L64
  constraint perpendicular L64 L65
  constraint perpendicular L49 L66
  constraint perpendicular L66 L67
  constraint perpendicular L67 L68
  constraint perpendicular L68 L69
  constraint perpendicular L69 L70
  constraint perpendicular L65 L71
  constraint perpendicular L71 L72
  constraint perpendicular L70 L73
  constraint perpendicular L75 L76
  constraint perpendicular L77 L78
  constraint perpendicular L79 L80
  constraint perpendicular L80 L81
  constraint horizontal L83
  constraint perpendicular L83 L84
  constraint perpendicular L84 L85
  constraint horizontal L87
  constraint horizontal L88
  constraint horizontal L89
  constraint perpendicular L87 L90
  constraint perpendicular L90 L91
  constraint perpendicular L88 L93
  constraint perpendicular L93 L94
  constraint perpendicular L89 L96
  constraint perpendicular L96 L97
  constraint coincident L0.end L115.start
  constraint perpendicular L0 L115
  constraint perpendicular L115 L116
  constraint coincident L0.start L117.end
  constraint vertical L118
  constraint perpendicular L120 L121
  constraint perpendicular L122 L139
  constraint perpendicular L122 L123
  constraint perpendicular L124 L139
  constraint perpendicular L125 L126
  constraint perpendicular L127 L144
  constraint perpendicular L128 L129
  constraint perpendicular L130 L144
  constraint collinear L131 L144
  constraint perpendicular L132 L133
  constraint perpendicular L134 L139
  constraint collinear L135 L139
  constraint coincident L137.end L139
  constraint perpendicular L137 L139
  constraint perpendicular L138 L139
  constraint collinear L139 L140
  constraint coincident L141.end L144
  constraint perpendicular L141 L144
  constraint collinear L144 L145
  constraint perpendicular L122 L146
  constraint horizontal L147
  constraint perpendicular L25 L148
  constraint perpendicular L125 L149
  constraint horizontal L150
  constraint perpendicular L36 L151
  constraint perpendicular L152 L153
  constraint perpendicular L153 L154
  constraint perpendicular L152 L155
  constraint perpendicular L156 L157
  constraint perpendicular L157 L158
  constraint perpendicular L156 L159
  constraint perpendicular L47 L160
  constraint perpendicular L160 L161
  constraint perpendicular L161 L162
  constraint perpendicular L162 L163
  measures "d170" distance of L50.end L51.end
  measures "d171" distance of L48.end L53.end
  measures "d172" distance of L53.end L54.end
  measures "d173" distance of L54.end L55.end
  measures "d174" distance of L55.end L56.end
  measures "d176" distance of L58.start L58.end
  measures "d177" distance of L58.end L59.end
  measures "d215" distance of L58.start L62.end
  measures "d216" distance of L49.start L66.end
  measures "d217" distance of L67.end L68.end
  measures "d218" distance of L68.end L69.end
  measures "d219" distance of L69.end L70.end
  measures "d220" distance of L65.end L71.end
  measures "d256" distance of L75.start L75.end
  measures "d257" angle of L76 L77
  measures "d258" distance of L76.end L77.end
  measures "d259" distance of L79.start L79.end
  measures "d260" distance of L79.end L80.end
  measures "d261" distance of L80.end L81.end
  measures "d313" distance of L84.end L85.end
  measures "d314" distance of L90.end L91.end
  measures "d315" distance of L93.end L94.end
  measures "d316" distance of L89.start L96.end
  measures "d317" distance of L96.end L97.end
  measures "d402" distance of L118.start L118.end
  measures "d522" distance of L122.start L122.end
  measures "d523" distance of L122.end L123.end
  measures "d525" distance of L125.start L125.end
  measures "d526" distance of L125.end L126.end
  measures "d529" distance of L131.end L128.start
  measures "d530" distance of L131.end L132.start
  measures "d531" distance of L128.start L128.end
  measures "d532" distance of L128.end L129.end
  measures "d533" distance of L129.end L130.end
  measures "d534" distance of L132.start L132.end
  measures "d535" distance of L132.end L133.end
  measures "d536" distance of L136.start L136.end
  measures "d539" distance of L141
  measures "d579" distance of L122.start L146.end
  measures "d580" distance of L146.end L147.end
  measures "d581" distance of L125.start L149.end
  measures "d582" distance of L149.end L150.end
  measures "d764" distance of L47.start L160.end
  measures "d765" distance of L160.end L161.end
  measures "d766" distance of L161.end L162.end
  measures "d767" distance of L162.end L163.end
extrude "Extrude19" add sketch "Sketch5" along normal blind 3 separate body contours L5 L6 L7 L8 L9 L10 L11 L12 L13 L14 L15 L16 L17 L18 L19 L20 L21 L22 L23 L24 L25 L26 L27 L28 L29 L30 L31 L32 L33 L34 L35 L36 L37 L38 L39 L40 L41 L42 L43 L44 L45 L46 L47 L48 L49 L50 L51 L52 L53 L54 L55 L56 L57 L58 L59 L60 L61 L62 L63 L64 L65 L66 L67 L68 L69 L70 L71 L72 L73 L74 L122 L123 L124 L125 L126 L127 L128 L129 L130 L131 L132 L133 L134 L135 L136 L137 L138 L139 L140 L141 L142 L143 L144 L145 L146 L147 L148 L149 L150 L151 L160 L161 L162 L163 L164 | L118 L119 L120 L121 makes body 19
ref_plane "WorkPlane5" through (-49.5, 51, 11.5) normal (0, 1, 0) x (-1, 0, 0)
sketch "Sketch6" plane through (0, 51, 0) normal (0, 1, 0) x (-1, 0, 0)
  line L0 (-68, 10) -> (-84, 10)
  line L1 (-39, 10) -> (-65, 10)
  line L2 (-10, 10) -> (-36, 10)
  line L3 (19, 10) -> (-7, 10)
  line L4 (48, 10) -> (22, 10)
  line L5 (77, 10) -> (51, 10)
  line L6 (93, 10) -> (80, 10)
  line L7 (93, 10) -> (93, -5)
  line L8 (80, 10) -> (80, 13)
  line L9 (51, 10) -> (51, 13)
  line L10 (51, 13) -> (48, 13)
  line L11 (48, 13) -> (48, 10)
  line L12 (36.5, -3) -> (36.5, 3)
  line L13 (33.5, -3) -> (36.5, -3)
  line L14 (33.5, 3) -> (33.5, -3)
  line L15 (36.5, 3) -> (33.5, 3)
  line L16 (59.5, -3) -> (59.5, -9)
  line L17 (62.5, -3) -> (59.5, -3)
  line L18 (62.5, -9) -> (62.5, -3)
  line L19 (59.5, -9) -> (62.5, -9)
  line L20 (79.5, -3) -> (79.5, -9)
  line L21 (82.5, -3) -> (79.5, -3)
  line L22 (82.5, -9) -> (82.5, -3)
  line L23 (79.5, -9) -> (82.5, -9)
  line L24 (19, 13) -> (19, 10)
  line L25 (22, 13) -> (19, 13)
  line L26 (22, 10) -> (22, 13)
  line L27 (-7, 10) -> (-7, 13)
  line L28 (-7, 13) -> (-10, 13)
  line L29 (-10, 13) -> (-10, 10)
  line L30 (-1.5, 3) -> (-1.5, -3)
  line L31 (1.5, 2.9851) -> (-1.5, 2.9851)
  line L32 (1.5, -3) -> (1.5, 3)
  line L33 (-1.5, -3) -> (1.5, -3)
  line L34 (-33.5, -3) -> (-33.5, 3)
  line L35 (-33.5, 2.9851) -> (-36.5, 2.9851)
  line L36 (-36.5, 3) -> (-36.5, -3)
  line L37 (-36.5, -3) -> (-33.5, -3)
  line L38 (-36, 10) -> (-36, 13)
  line L39 (-36, 13) -> (-39, 13)
  line L40 (-39, 13) -> (-39, 10)
  line L41 (-65, 10) -> (-65, 13)
  line L42 (-65, 13) -> (-68, 13)
  line L43 (-68, 13) -> (-68, 10)
  line L44 (-82.5, -3) -> (-79.5, -3)
  line L45 (-82.5, -3) -> (-82.5, -9)
  line L46 (-79.5, -9) -> (-82.5, -9)
  line L47 (-79.5, -3) -> (-79.5, -9)
  line L48 (-62.5, -3) -> (-62.5, -9)
  line L49 (-59.5, -3) -> (-62.5, -3)
  line L50 (-59.5, -9) -> (-59.5, -3)
  line L51 (-62.5, -9) -> (-59.5, -9)
  arc A0 (88, -10) -> (93, -5) centre (88, -5) ccw
  line L52 (80, 13) -> (77, 13)
  line L53 (77, 13) -> (77, 10)
  line L54 (-84, 10) -> (-84, 1.5)
  line L55 (85, -4.5) -> (88, -4.5)
  line L56 (85, -1.5) -> (85, -4.5)
  line L57 (88, -1.5) -> (85, -1.5)
  line L58 (88, -4.5) -> (88, -1.5)
  line L59 (-84, -1.5) -> (-87, -1.5)
  line L60 (-87, -1.5) -> (-87, 1.5)
  line L61 (-84, 1.5) -> (-87, 1.5)
  line L62 (-84, -1.5) -> (-84, -10)
  line L63 (-84, -10) -> (88, -10)
  dimension "d160" = 5
  constraint coincident L8.end L52.start
  constraint coincident L5.start L53.end
  constraint perpendicular L5 L53
  constraint coincident L62.end L63.start
  constraint tangent A0 L63
  measures "d160" radius of A0
extrude "Extrude20" add sketch "Sketch6" along normal blind 3 separate body makes body 20
ref_plane "WorkPlane6" through (-3, 54, 1.5) normal (0, 1, 0) x (-1, 0, 0)
sketch "Sketch7" plane through (0, 54, 0) normal (0, 1, 0) x (0, 0, 1)
  circle A0 centre (-6, 81) radius 9
  line L0 (-9, 82.5) -> (-9, 79.5)
  line L1 (-3, 82.5) -> (-9, 82.5)
  line L2 (-3, 79.5) -> (-3, 82.5)
  line L3 (-9, 79.5) -> (-3, 79.5)
  line L4 (-3, 62.5) -> (-9, 62.5)
  line L5 (-3, 62.5) -> (-3, 59.5)
  line L6 (-9, 59.5) -> (-3, 59.5)
  line L7 (-9, 62.5) -> (-9, 59.5)
  circle A1 centre (-6, 61) radius 9
  circle A2 centre (0, 35) radius 15
  line L8 (-3, 36.5) -> (3, 36.5)
  line L9 (-3, 33.5) -> (-3, 36.5)
  line L10 (3, 33.5) -> (-3, 33.5)
  line L11 (3, 36.5) -> (3, 33.5)
  circle A3 centre (0, 0) radius 15
  circle A4 centre (0, -35) radius 15
  circle A5 centre (-6, -61) radius 9
  circle A6 centre (-6, -81) radius 9
  line L12 (-3, -62.5) -> (-3, -59.5)
  line L13 (-9, -59.5) -> (-3, -59.5)
  line L14 (-3, -62.5) -> (-9, -62.5)
  line L15 (-9, -62.5) -> (-9, -59.5)
  line L16 (-3, -36.5) -> (3, -36.5)
  line L17 (-3, -33.5) -> (-3, -36.5)
  line L18 (3, -33.5) -> (-3, -33.5)
  line L19 (3, -36.5) -> (3, -33.5)
  line L20 (3, -1.5) -> (-3, -1.5)
  line L21 (-3, -1.5) -> (-3, 1.5)
  line L22 (-3, 1.5) -> (3, 1.5)
  line L23 (3, 1.5) -> (3, -1.5)
  line L24 (-9, -79.5) -> (-3, -79.5)
  line L25 (-3, -79.5) -> (-3, -82.5)
  line L26 (-3, -82.5) -> (-9, -82.5)
  line L27 (-9, -82.5) -> (-9, -79.5)
  point P0 (-9, -59.5)
extrude "Extrude21" add sketch "Sketch7" along normal blind 3 separate body contours A0 makes body 21
extrude "Extrude22" add sketch "Sketch7" along normal blind 3 separate body contours A1 makes body 22
extrude "Extrude23" add sketch "Sketch7" along normal blind 3 separate body contours A2 makes body 23
extrude "Extrude24" add sketch "Sketch7" along normal blind 3 separate body contours A3 makes body 24
extrude "Extrude25" add sketch "Sketch7" along normal blind 3 separate body contours A4 makes body 25
extrude "Extrude26" add sketch "Sketch7" along normal blind 3 separate body contours A5 makes body 26
extrude "Extrude27" add sketch "Sketch7" along normal blind 3 separate body contours A6 makes body 27
ref_plane "WorkPlane7" through (-35, 57, 0) normal (0, 1, 0) x (0, 0, 1)